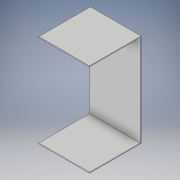
# Autodesk Inventor part: Platinenhalter
Saved by Autodesk Inventor 2017.3 (Build 213256000, 256)
## iProperties
Part Number: Platinenhalter
Material: Generisch
Document SubType Name: Modeling
Designer: Nils
Density: 1 g/cm^3
Appearance: Vorgabe
Author: Nils
Autodesk Inventor part; units mm, degrees
ref_plane "YZ Plane" through (0, 0, 0) normal (1, 0, 0) x (0, 1, 0)
ref_plane "XZ Plane" through (0, 0, 0) normal (0, 1, 0) x (-1, 0, 0)
ref_plane "XY Plane" through (0, 0, 0) normal (0, 0, 1) x (1, 0, 0)
sketch "Skizze1" plane through (0, 0, 0) normal (1, 0, 0) x (0, 1, 0)
  line L0 (-45.75, 82.5) -> (45.75, 82.5)
  line L1 (45.75, 82.5) -> (45.75, -82.5)
  line L2 (45.75, -82.5) -> (-45.75, -82.5)
  line L3 (-45.75, 81) -> (44.25, 81)
  line L4 (44.25, 81) -> (44.25, -81)
  line L5 (44.25, -81) -> (-45.75, -81)
  line L6 (-45.75, -82.5) -> (-45.75, -81)
  line L7 (-45.75, 81) -> (-45.75, 82.5)
  point P0 (0, 0)
  point P1 (0, 82.5)
  point P2 (45.75, 0)
  dimension "d0" = 1.5
  dimension "d1" = 1.5
  dimension "d2" = 1.5
  dimension "d3" = 90
  dimension "d4" = 165
  constraints: 16 end point, 4 parallel, 2 horizontal, 2 midpoint, 2 perpendicular, 2 vertical alignment, 1 horizontal alignment
  measures "d0" distance of L3.start L0.start
  measures "d1" distance of L2.end L5.end
  measures "d2" distance between parallel lines of L1 L4
  measures "d3" distance of L3.start L3.end
  measures "d4" distance of L0.end L1.end
extrude "Extrusion1" add sketch "Skizze1" along normal mid plane 90
